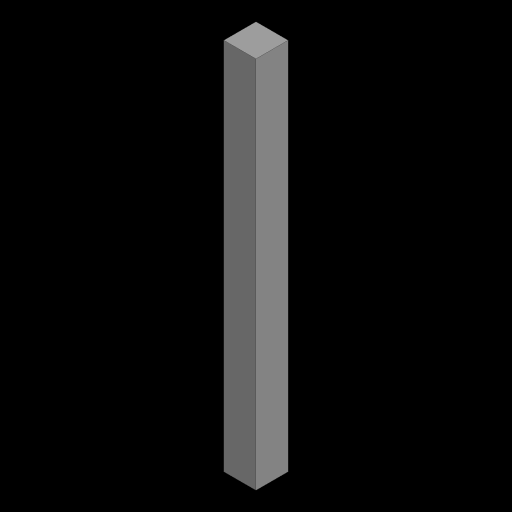
# Autodesk Inventor part: rp_lever
Saved by Autodesk Inventor 2023 (Build 270158000, 158)
## iProperties
Created: 2024-07-04
Part Number: rp_lever
Material: 일반
Document SubType Name: Modeling
Designer: OMS55
Density: 1 g/cm^3
Appearance: 기본값
Mass: 8.64051 g
Surface Area: 37.7708 cm^2
Volume: 8.64051 cm^3
Author: OMS55
Autodesk Inventor part; units mm, degrees
ref_plane "YZ Plane" through (0, 0, 0) normal (1, 0, 0) x (0, 1, 0)
ref_plane "XZ Plane" through (0, 0, 0) normal (0, 1, 0) x (-1, 0, 0)
ref_plane "XY Plane" through (0, 0, 0) normal (0, 0, 1) x (1, 0, 0)
sketch "스케치1" plane through (0, 0, 0) normal (0, 1, 0) x (-1, 0, 0)
  circle A0 centre (0, 0) radius 3.1
  line L0 (2.15, 2.15) -> (-2.15, 2.15)
  line L1 (-2.15, 2.15) -> (-2.15, -2.15)
  line L2 (-2.15, -2.15) -> (2.15, -2.15)
  line L3 (2.15, -2.15) -> (2.15, 2.15)
  point P0 (2.15, 0)
  point P1 (0, 2.15)
  dimension "d0" = 6.2
  dimension "d7" = 4.3
  dimension "d8" = 4.3
  constraints: 8 end point, 2 midpoint, 1 centre point, 1 coincident, 1 horizontal, 1 horizontal alignment, 1 parallel, 1 perpendicular, 1 vertical alignment
  measures "d0" diameter of A0
  measures "d7" distance of L0.start L0.end
  measures "d8" distance of L0.end L1.end
extrude "돌출1" add sketch "스케치1" along normal blind 50 contours L3 L2 L1 L0
